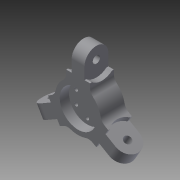
# Autodesk Inventor part: hub
Saved by Autodesk Inventor 2014 SP2 (Build 180246200, 246)
## iProperties
Created: 2016-12-02
Part Number: hub
Material: Generic
Document SubType Name: Modeling
Designer: Justin B
Density: 1 g/cm^3
Appearance: Default
Author: Justin B
Autodesk Inventor part; units mm, degrees
ref_plane "YZ Plane" through (0, 0, 0) normal (1, 0, 0) x (0, 1, 0)
ref_plane "XZ Plane" through (0, 0, 0) normal (0, 1, 0) x (-1, 0, 0)
ref_plane "XY Plane" through (0, 0, 0) normal (0, 0, 1) x (1, 0, 0)
sketch "Sketch1" plane through (0, 0, 0) normal (0, 1, 0) x (-1, 0, 0)
  circle A0 centre (0, 0) radius 25
  line L0 (0, 0) -> (0, 25) construction
  line L1 (0, 0) -> (21.6506, -12.5) construction
  line L2 (0, 0) -> (-21.6506, -12.5) construction
  line L3 (13, 21.3542) -> (13, 26.3542)
  line L4 (13, 26.3542) -> (-13, 26.3542)
  line L5 (-13, 26.3542) -> (-13, 21.3542)
  line L6 (7, 26.3542) -> (7, 56.3542)
  line L7 (7, 56.3542) -> (-7, 56.3542)
  line L8 (-7, 56.3542) -> (-7, 26.3542)
  dimension "d0" = 50
  dimension "d1" = 120
  dimension "d2" = 120
  dimension "d3" = 26
  dimension "d4" = 5
  dimension "d5" = 30
  dimension "d6" = 14
  constraints: 18 end point, 5 point on circle, 3 parallel, 3 perpendicular, 2 point on line, 1 centre point, 1 coincident, 1 vertical, 2 other
  measures "d0" diameter of A0
  measures "d1" angle of L0 L1
  measures "d2" angle of L2 L0
  measures "d3" distance between parallel lines of L5 L3
  measures "d4" distance of L3.start L3.end
  measures "d5" distance of L6.start L6.end
  measures "d6" distance of L6.end L7.end
extrude "Extrusion1" add sketch "Sketch1" along normal blind 26
sketch "Sketch2" plane through (7, 0, 56.3542) normal (1, 0, 0) x (0, 0, -1)
  line L0 (0, 0) -> (0, 26) projected
  circle A0 centre (13, 13) radius 4
  point P0 (56.3542, 0)
  point P1 (0, 13)
  dimension "d12" = 8
  dimension "d13" = 13
  constraints: 1 centre point, 1 horizontal alignment, 1 midpoint
  measures "d12" diameter of A0
  measures "d13" distance from line of L0 A0.centre
extrude "Extrusion2" cut sketch "Sketch2" against normal up to next
fillet "Fillet1" radius 13 2 edges at (0, 26, 56.3542) (0, 0, 56.3542)
sketch "Sketch3" plane through (-7, 0, 26.3542) normal (-1, 0, 0) x (0, 0, 1)
  line L0 (0, 26) -> (17, 26) projected
  line L1 (0, 0) -> (0, 26) projected
  line L2 (0, 0) -> (17, 0) projected
  circle A0 centre (17, 13) radius 4 projected
  arc A1 (0, 13) -> (6.0455, 0) centre (17, 13) ccw
  arc A2 (6.0455, 26) -> (0, 13) centre (17, 13) ccw
  line L3 (6.0455, 26) -> (0, 26)
  line L4 (0, 0) -> (6.0455, 0)
  arc A3 (17, 0) -> (17, 26) centre (17, 13) ccw projected
  circle A4 centre (17, 13) radius 13 construction
  line L5 (4, 2.0455) -> (4, 23.9545) construction
  line L6 (4, 23.9545) -> (4, 26)
  line L7 (4, 2.0455) -> (4, 0)
  point P0 (-26.3542, 0)
  constraints: 10 end point, 6 point on circle, 3 centre point, 3 coincident, 3 perpendicular, 2 collinear, 2 point on line, 1 concentric, 1 midpoint, 1 tangent
extrude "Extrusion3" add sketch "Sketch3" along normal up to surface (6 mm away) contours L0 L6 A2 L1 | A1 L7 L2 L1
mirror "Mirror1" about plane through (0, 0, 0) normal (1, 0, 0) of "Extrusion3"
fillet "Fillet2" radius 10 2 edges at (-13, 13, 21.3542) (13, 13, 21.3542)
pattern_circular "Circular Pattern2" count 3 over 360 about axis through (0, -10, 0) along (0, 1, 0) of "Extrusion1", "Fillet2", "Extrusion3", "Mirror1", "Extrusion2", "Fillet1"
sketch "Sketch4" plane through (0, 26, 0) normal (0, 1, 0) x (1, 0, 0)
  arc A0 (-24.5338, -4.8055) -> (-16.4286, -18.8442) centre (0, 0) ccw projected
  arc A1 (8.1052, 23.6496) -> (-8.1052, 23.6496) centre (0, 0) ccw projected
  circle A2 centre (0, 0) radius 14 construction
  circle A3 centre (0, 14) radius 2
  dimension "d23" = 28
  dimension "d24" = 4
  constraints: 2 vertical alignment, 1 centre point, 1 coincident, 2 other
  measures "d24" diameter of A3
extrude "Extrusion4" cut sketch "Sketch4" against normal up to next
pattern_circular "Circular Pattern3" count 6 over 360 about axis through (0, -10, 0) along (0, 1, 0) of "Extrusion4"
sketch "Sketch6" plane through (0, 0, 0) normal (0, -1, 0) x (1, 0, 0)
  circle A0 centre (12.1244, -7) radius 2 projected
  circle A1 centre (12.1244, 7) radius 2 projected
  circle A2 centre (0, 14) radius 2 projected
  circle A3 centre (-12.1244, 7) radius 2 projected
  circle A4 centre (-12.1244, -7) radius 2 projected
  circle A5 centre (0, -14) radius 2 projected
  arc A6 (-16.4286, 18.8442) -> (-24.5338, 4.8055) centre (0, 0) ccw projected
  circle A7 centre (0, 0) radius 20
  dimension "d33" = 40
  constraints: 1 centre point, 1 coincident
  measures "d33" diameter of A7
extrude "Extrusion6" cut sketch "Sketch6" against normal blind 10
body "Solid1"
